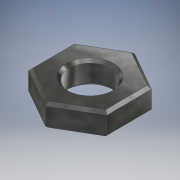
# Autodesk Inventor part: TuercaManzana
Saved by Autodesk Inventor 2017 (Build 210142000, 142)
## iProperties
Created: 2016-06-28
Part Number: TuercaManzana
Material: Steel
Document SubType Name: Modeling
Designer: YeseF
Density: 7.85 g/cm^3
Appearance: Steel Galvanized
Author: YeseF
Autodesk Inventor part; units mm, degrees
ref_plane "YZ Plane" through (0, 0, 0) normal (1, 0, 0) x (0, 1, 0)
ref_plane "XZ Plane" through (0, 0, 0) normal (0, 1, 0) x (-1, 0, 0)
ref_plane "XY Plane" through (0, 0, 0) normal (0, 0, 1) x (1, 0, 0)
sketch "Sketch1" plane through (0, 0, 0) normal (0, 0, 1) x (1, 0, 0)
  circle A0 centre (0, 0) radius 4.51
  line L0 (-0.0588, 9.8148) -> (8.4705, 4.9583)
  line L1 (8.4705, 4.9583) -> (8.5292, -4.8565)
  line L2 (8.5292, -4.8565) -> (0.0588, -9.8148)
  line L3 (0.0588, -9.8148) -> (-8.4705, -4.9583)
  line L4 (-8.4705, -4.9583) -> (-8.5292, 4.8565)
  line L5 (-8.5292, 4.8565) -> (-0.0588, 9.8148)
  dimension "d0" = 9.02
  dimension "d1" = 8.5
  constraints: 12 end point, 2 coincident, 1 centre point, 13 other
  measures "d0" diameter of A0
  measures "d1" distance from line of point (0, 0) L5
extrude "Extrusion1" add sketch "Sketch1" along normal blind 5
chamfer "Chamfer1" distance 0.6 angle 45 14 edges at (-4.294, 7.3356, 5) (-8.4998, -0.0509, 5) (-4.2058, -7.3865, 5) (4.294, -7.3356, 5) (8.4998, 0.0509, 5) (4.2058, 7.3865, 5) (-4.2058, -7.3865, 0) (4.294, -7.3356, 0) (8.4998, 0.0509, 0) (4.2058, 7.3865, 0) (-4.294, 7.3356, 0) (-8.4998, -0.0509, 0) (-4.51, 0, 5) (-4.51, 0, 0)
body "Solid1"
